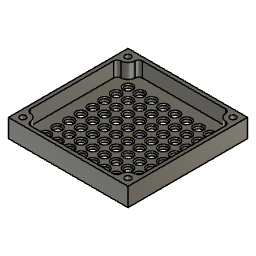
LED MATRIX GRILL (Autodesk Fusion 360 design; units mm, degrees)
Autodesk Fusion 360 part; units mm, degrees
sketch "Sketch1" plane through (0, 0, 0) normal (0, 0, 1) x (1, 0, 0)
  line L0 (32.4, 32.4) -> (-32.4, 32.4)
  line L1 (-32.4, 32.4) -> (-32.4, -32.4)
  line L2 (-32.4, -32.4) -> (32.4, -32.4)
  line L3 (32.4, -32.4) -> (32.4, 32.4)
  line L4 (32.4, 32.4) -> (-32.4, -32.4) construction
  line L5 (-32.4, 32.4) -> (32.4, -32.4) construction
  line L6 (28.5, -28.5) -> (-28.5, -28.5)
  line L7 (-28.5, -28.5) -> (-28.5, 28.5)
  line L8 (-28.5, 28.5) -> (28.5, 28.5)
  line L9 (28.5, 28.5) -> (28.5, -28.5)
  line L10 (28.5, -28.5) -> (-28.5, 28.5) construction
  circle A0 centre (28.5, 28.5) radius 1.6
  circle A1 centre (-28.5, 28.5) radius 1.6
  circle A2 centre (-28.5, -28.5) radius 1.6
  circle A3 centre (28.5, -28.5) radius 1.6
  line L11 (25.6, 25.6) -> (-25.6, 25.6)
  line L12 (-25.6, 25.6) -> (-25.6, -25.6)
  line L13 (-25.6, -25.6) -> (25.6, -25.6)
  line L14 (25.6, -25.6) -> (25.6, 25.6)
  line L15 (25.6, 25.6) -> (-25.6, -25.6) construction
  line L16 (-25.6, 25.6) -> (25.6, -25.6) construction
  line L17 (22.2, 22.2) -> (-22.2, -22.2) construction
  line L18 (-22.2, 22.2) -> (22.2, -22.2) construction
  line L19 (15.9, 15.9) -> (-15.9, -15.9) construction
  line L20 (-15.9, 15.9) -> (15.9, -15.9) construction
  line L21 (22.3, 22.3) -> (-22.3, 22.3)
  line L22 (-22.3, 22.3) -> (-22.3, -22.3)
  line L23 (-22.3, -22.3) -> (22.3, -22.3)
  line L24 (22.3, -22.3) -> (22.3, 22.3)
  line L25 (22.3, 22.3) -> (-22.3, -22.3) construction
  line L26 (-22.3, 22.3) -> (22.3, -22.3) construction
  line L27 (-22.3, 22.3) -> (-15.9286, 22.3)
  line L28 (-15.9286, 22.3) -> (-15.9286, -22.3)
  line L29 (-15.9286, -22.3) -> (-22.3, -22.3)
  line L30 (-22.3, -22.3) -> (-22.3, 22.3)
  line L31 (-15.9286, 22.3) -> (-9.5571, 22.3)
  line L32 (-9.5571, 22.3) -> (-9.5571, -22.3)
  line L33 (-9.5571, -22.3) -> (-15.9286, -22.3)
  line L34 (-15.9286, -22.3) -> (-15.9286, 22.3)
  line L35 (-9.5571, 22.3) -> (-3.1857, 22.3)
  line L36 (-3.1857, 22.3) -> (-3.1857, -22.3)
  line L37 (-3.1857, -22.3) -> (-9.5571, -22.3)
  line L38 (-9.5571, -22.3) -> (-9.5571, 22.3)
  line L39 (-3.1857, 22.3) -> (3.1857, 22.3)
  line L40 (3.1857, 22.3) -> (3.1857, -22.3)
  line L41 (3.1857, -22.3) -> (-3.1857, -22.3)
  line L42 (-3.1857, -22.3) -> (-3.1857, 22.3)
  line L43 (3.1857, 22.3) -> (9.5571, 22.3)
  line L44 (9.5571, 22.3) -> (9.5571, -22.3)
  line L45 (9.5571, -22.3) -> (3.1857, -22.3)
  line L46 (3.1857, -22.3) -> (3.1857, 22.3)
  line L47 (9.5571, 22.3) -> (15.9286, 22.3)
  line L48 (15.9286, 22.3) -> (15.9286, -22.3)
  line L49 (15.9286, -22.3) -> (9.5571, -22.3)
  line L50 (9.5571, -22.3) -> (9.5571, 22.3)
  line L51 (22.3, 22.3) -> (-22.3, 22.3)
  line L52 (-22.3, 22.3) -> (-22.3, 15.9286)
  line L53 (-22.3, 15.9286) -> (22.3, 15.9286)
  line L54 (22.3, 15.9286) -> (22.3, 22.3)
  line L55 (-22.3, 15.9286) -> (22.3, 15.9286)
  line L56 (22.3, 15.9286) -> (22.3, 9.5571)
  line L57 (22.3, 9.5571) -> (-22.3, 9.5571)
  line L58 (-22.3, 9.5571) -> (-22.3, 15.9286)
  line L59 (-22.3, 9.5571) -> (22.3, 9.5571)
  line L60 (22.3, 9.5571) -> (22.3, 3.1857)
  line L61 (22.3, 3.1857) -> (-22.3, 3.1857)
  line L62 (-22.3, 3.1857) -> (-22.3, 9.5571)
  line L63 (-22.3, 3.1857) -> (22.3, 3.1857)
  line L64 (22.3, 3.1857) -> (22.3, -3.1857)
  line L65 (22.3, -3.1857) -> (-22.3, -3.1857)
  line L66 (-22.3, -3.1857) -> (-22.3, 3.1857)
  line L67 (-22.3, -3.1857) -> (22.3, -3.1857)
  line L68 (22.3, -3.1857) -> (22.3, -9.5571)
  line L69 (22.3, -9.5571) -> (-22.3, -9.5571)
  line L70 (-22.3, -9.5571) -> (-22.3, -3.1857)
  line L71 (-22.3, -9.5571) -> (22.3, -9.5571)
  line L72 (22.3, -9.5571) -> (22.3, -15.9286)
  line L73 (22.3, -15.9286) -> (-22.3, -15.9286)
  line L74 (-22.3, -15.9286) -> (-22.3, -9.5571)
  circle A4 centre (-22.2, 22.2) radius 2
  circle A5 centre (-15.9286, 22.3) radius 2
  circle A6 centre (-9.5571, 22.3) radius 2
  circle A7 centre (-3.1857, 22.3) radius 2
  circle A8 centre (3.1857, 22.3) radius 2
  circle A9 centre (9.5571, 22.3) radius 2
  circle A10 centre (15.9286, 22.3) radius 2
  circle A11 centre (22.2, 22.2) radius 2
  circle A12 centre (-22.3, 15.9286) radius 2
  circle A13 centre (-15.9286, 15.9286) radius 2
  circle A14 centre (-9.5571, 15.9286) radius 2
  circle A15 centre (-3.1857, 15.9286) radius 2
  circle A16 centre (3.1857, 15.9286) radius 2
  circle A17 centre (9.5571, 15.9286) radius 2
  circle A18 centre (15.9286, 15.9286) radius 2
  circle A19 centre (22.3, 15.9286) radius 2
  circle A20 centre (22.3, 9.5571) radius 2
  circle A21 centre (15.9286, 9.5571) radius 2
  circle A22 centre (9.5571, 9.5571) radius 2
  circle A23 centre (3.1857, 9.5571) radius 2
  circle A24 centre (-3.1857, 9.5571) radius 2
  circle A25 centre (-9.5571, 9.5571) radius 2
  circle A26 centre (-15.9286, 9.5571) radius 2
  circle A27 centre (-22.3, 9.5571) radius 2
  circle A28 centre (-22.3, 3.1857) radius 2
  circle A29 centre (-15.9286, 3.1857) radius 2
  circle A30 centre (-9.5571, 3.1857) radius 2
  circle A31 centre (-3.1857, 3.1857) radius 2
  circle A32 centre (3.1857, 3.1857) radius 2
  circle A33 centre (9.5571, 3.1857) radius 2
  circle A34 centre (15.9286, 3.1857) radius 2
  circle A35 centre (22.3, 3.1857) radius 2
  circle A36 centre (22.3, -3.1857) radius 2
  circle A37 centre (15.9286, -3.1857) radius 2
  circle A38 centre (9.5571, -3.1857) radius 2
  circle A39 centre (3.1857, -3.1857) radius 2
  circle A40 centre (-3.1857, -3.1857) radius 2
  circle A41 centre (-9.5571, -3.1857) radius 2
  circle A42 centre (-15.9286, -3.1857) radius 2
  circle A43 centre (-22.3, -3.1857) radius 2
  circle A44 centre (-22.3, -9.5571) radius 2
  circle A45 centre (-15.9286, -9.5571) radius 2
  circle A46 centre (-9.5571, -9.5571) radius 2
  circle A47 centre (-3.1857, -9.5571) radius 2
  circle A48 centre (3.1857, -9.5571) radius 2
  circle A49 centre (9.5497, -9.5497) radius 2
  circle A50 centre (15.9286, -9.5571) radius 2
  circle A51 centre (22.3, -9.5571) radius 2
  circle A52 centre (-22.3, -15.9286) radius 2
  circle A53 centre (-22.3, -22.3) radius 2
  circle A54 centre (-15.9286, -22.3) radius 2
  circle A55 centre (-15.9286, -15.9286) radius 2
  circle A56 centre (-9.5571, -15.9286) radius 2
  circle A57 centre (-9.5571, -22.3) radius 2
  circle A58 centre (-3.1857, -15.9286) radius 2
  circle A59 centre (-3.1857, -22.3) radius 2
  circle A60 centre (3.1857, -15.9286) radius 2
  circle A61 centre (3.1857, -22.3) radius 2
  circle A62 centre (9.5571, -15.9286) radius 2
  circle A63 centre (9.5571, -22.3) radius 2
  circle A64 centre (15.9314, -15.9314) radius 2
  circle A65 centre (15.9286, -22.3) radius 2
  circle A66 centre (22.3, -15.9286) radius 2
  circle A67 centre (22.3, -22.3) radius 2
  dimension "d1" = 64.8
  dimension "d2" = 64.8
  dimension "d3" = 57
  dimension "d4" = 57
  dimension "d5" = 3.2
  dimension "d6" = 3.2
  dimension "d7" = 3.2
  dimension "d8" = 3.2
  dimension "d9" = 51.2
  dimension "d10" = 51.2
  dimension "d11" = 44.4
  dimension "d12" = 44.4
  dimension "d15" = 44.6
  dimension "d16" = 44.6
  dimension "d17" = 6.3714
  dimension "d18" = 44.6
  dimension "d19" = 6.3714
  dimension "d20" = 6.3714
  dimension "d21" = 6.3714
  dimension "d22" = 6.3714
  dimension "d23" = 6.3714
  dimension "d24" = 6.3714
  dimension "d25" = 6.3714
  dimension "d26" = 6.3714
  dimension "d27" = 6.3714
  dimension "d28" = 6.3714
  dimension "d29" = 6.3714
  dimension "d30" = 4
  dimension "d31" = 4
  dimension "d32" = 4
  dimension "d33" = 4
  dimension "d34" = 4
  dimension "d35" = 4
  dimension "d36" = 4
  dimension "d37" = 4
  dimension "d38" = 4
  dimension "d39" = 4
  dimension "d40" = 4
  dimension "d41" = 4
  dimension "d42" = 4
  dimension "d43" = 4
  dimension "d44" = 4
  dimension "d45" = 4
  dimension "d46" = 4
  dimension "d47" = 4
  dimension "d48" = 4
  dimension "d49" = 4
  dimension "d50" = 4
  dimension "d51" = 4
  dimension "d52" = 4
  dimension "d53" = 4
  dimension "d54" = 4
  dimension "d55" = 4
  dimension "d56" = 4
  dimension "d57" = 4
  dimension "d58" = 4
  dimension "d59" = 4
  dimension "d60" = 4
  dimension "d61" = 4
  dimension "d62" = 4
  dimension "d63" = 4
  dimension "d64" = 4
  dimension "d65" = 4
  dimension "d66" = 4
  dimension "d67" = 4
  dimension "d68" = 4
  dimension "d69" = 4
  dimension "d70" = 4
  dimension "d71" = 4
  dimension "d72" = 4
  dimension "d73" = 4
  dimension "d74" = 4
  dimension "d75" = 4
  dimension "d76" = 4
  dimension "d77" = 4
  dimension "d78" = 4
  dimension "d79" = 4
  dimension "d80" = 4
  dimension "d81" = 4
  dimension "d82" = 4
  dimension "d83" = 4
  dimension "d84" = 4
  dimension "d85" = 4
  dimension "d86" = 4
  dimension "d87" = 4
  dimension "d88" = 4
  dimension "d89" = 4
  dimension "d90" = 4
  dimension "d91" = 4
  dimension "d92" = 4
  dimension "d93" = 4
  constraint horizontal L0
  constraint perpendicular L0 L1
  constraint parallel L0 L2
  constraint parallel L1 L3
  constraint coincident L4 origin
  constraint coincident L5 origin
  constraint horizontal L6
  constraint perpendicular L6 L7
  constraint parallel L6 L8
  constraint parallel L7 L9
  constraint coincident L10 origin
  constraint coincident L8.end L9.start
  constraint coincident L7.end L8.start
  constraint coincident L6.end L7.start
  constraint coincident L6.start L9.end
  constraint horizontal L11
  constraint perpendicular L11 L12
  constraint parallel L11 L13
  constraint parallel L12 L14
  constraint coincident L15 origin
  constraint coincident L16 origin
  constraint coincident L17 origin
  constraint coincident L18 origin
  constraint coincident L19 origin
  constraint coincident L20 origin
  constraint horizontal L21
  constraint perpendicular L21 L22
  constraint parallel L21 L23
  constraint parallel L22 L24
  constraint coincident L25 origin
  constraint coincident L26 origin
  constraint horizontal L27
  constraint vertical L28
  constraint horizontal L29
  constraint vertical L30
  constraint horizontal L31
  constraint vertical L32
  constraint horizontal L33
  constraint vertical L34
  constraint horizontal L35
  constraint vertical L36
  constraint horizontal L37
  constraint vertical L38
  constraint horizontal L39
  constraint vertical L40
  constraint horizontal L41
  constraint vertical L42
  constraint horizontal L43
  constraint vertical L44
  constraint horizontal L45
  constraint vertical L46
  constraint horizontal L47
  constraint vertical L48
  constraint horizontal L49
  constraint vertical L50
  constraint horizontal L51
  constraint vertical L52
  constraint horizontal L53
  constraint vertical L54
  constraint horizontal L55
  constraint vertical L56
  constraint horizontal L57
  constraint vertical L58
  constraint horizontal L59
  constraint vertical L60
  constraint horizontal L61
  constraint vertical L62
  constraint horizontal L63
  constraint vertical L64
  constraint horizontal L65
  constraint vertical L66
  constraint horizontal L67
  constraint vertical L68
  constraint horizontal L69
  constraint vertical L70
  constraint horizontal L71
  constraint vertical L72
  constraint horizontal L73
  constraint vertical L74
  constraint coincident L18.start A4.centre
  constraint coincident L27.end L28.start
  constraint coincident L31.end L32.start
  constraint coincident L35.end L36.start
  constraint coincident L39.end L40.start
  constraint coincident L43.end L44.start
  constraint coincident L47.end L48.start
  constraint coincident L17.start A11.centre
  constraint coincident L52.end L53.start
  constraint coincident L28 A13.centre
  constraint coincident L26 A13.centre
  constraint coincident L55 A14.centre
  constraint coincident L32 A14.centre
  constraint coincident L55 A15.centre
  constraint coincident L42 A15.centre
  constraint coincident L40 A16.centre
  constraint coincident L53 A16.centre
  constraint coincident L53 A17.centre
  constraint coincident L50 A17.centre
  constraint coincident L48 A18.centre
  constraint coincident L53 A18.centre
  constraint coincident L53.end L54.start
  constraint coincident L56.end L57.start
  constraint coincident L48 A21.centre
  constraint coincident L57 A21.centre
  constraint coincident L50 A22.centre
  constraint coincident L57 A22.centre
  constraint coincident L46 A23.centre
  constraint coincident L57 A23.centre
  constraint coincident L42 A24.centre
  constraint coincident L59 A24.centre
  constraint coincident L38 A25.centre
  constraint coincident L16 A25.centre
  constraint coincident L57 A26.centre
  constraint coincident L28 A26.centre
  constraint coincident L57.end L58.start
  constraint coincident L61.end L62.start
  constraint coincident L34 A29.centre
  constraint coincident L61 A29.centre
  constraint coincident L32 A30.centre
  constraint coincident L63 A30.centre
  constraint coincident L61 A31.centre
  constraint coincident L42 A31.centre
  constraint coincident L17 A32.centre
  constraint coincident L46 A32.centre
  constraint coincident L61 A33.centre
  constraint coincident L44 A33.centre
  constraint coincident L61 A34.centre
  constraint coincident L48 A34.centre
  constraint coincident L60.end L61.start
  constraint coincident L64.end L65.start
  constraint coincident L48 A37.centre
  constraint coincident L67 A37.centre
  constraint coincident L50 A38.centre
  constraint coincident L65 A38.centre
  constraint coincident L67 A39.centre
  constraint coincident L16 A39.centre
  constraint coincident L65 A40.centre
  constraint coincident L42 A40.centre
  constraint coincident L32 A41.centre
  constraint coincident L65 A41.centre
  constraint coincident L34 A42.centre
  constraint coincident L65 A42.centre
  constraint coincident L65.end L66.start
  constraint coincident L69.end L70.start
  constraint coincident L28 A45.centre
  constraint coincident L71 A45.centre
  constraint coincident L71 A46.centre
  constraint coincident L38 A46.centre
  constraint coincident L42 A47.centre
  constraint coincident L71 A47.centre
  constraint coincident L46 A48.centre
  constraint coincident L71 A48.centre
  constraint coincident L16 A49.centre
  constraint coincident L71 A50.centre
  constraint coincident L48 A50.centre
  constraint coincident L68.end L69.start
  constraint coincident L73.end L74.start
  constraint coincident L22.end L23.start
  constraint coincident L28.end L29.start
  constraint coincident L28 A55.centre
  constraint coincident L73 A55.centre
  constraint coincident L38 A56.centre
  constraint coincident L73 A56.centre
  constraint coincident L32.end L33.start
  constraint coincident L42 A58.centre
  constraint coincident L73 A58.centre
  constraint coincident L36.end L37.start
  constraint coincident L46 A60.centre
  constraint coincident L73 A60.centre
  constraint coincident L40.end L41.start
  constraint coincident L44 A62.centre
  constraint coincident L73 A62.centre
  constraint coincident L44.end L45.start
  constraint coincident L18 A64.centre
  constraint coincident L48.end L49.start
  constraint coincident L72.end L73.start
  constraint coincident L23.end L24.start
  measures "d1" distance of L1.end L2.end
  measures "d2" distance of L0.end L1.end
  measures "d3" distance of L7.end L8.end
  measures "d4" distance of L6.end L7.end
  measures "d5" diameter of A0
  measures "d6" diameter of A1
  measures "d7" diameter of A2
  measures "d8" diameter of A3
  measures "d9" distance of L12.end L13.end
  measures "d10" distance of L11.end L12.end
  measures "d11" distance of L17.end L18.end
  measures "d12" distance of L18.start L17.end
  measures "d15" distance of L22.end L23.end
  measures "d16" distance of L21.end L22.end
  measures "d17" distance of L21.end L27.end
  measures "d18" distance of L21.end L22.end
  measures "d19" distance of L27.end L31.end
  measures "d20" distance of L31.end L35.end
  measures "d21" distance of L35.end L39.end
  measures "d22" distance of L39.end L43.end
  measures "d23" distance of L43.end L47.end
  measures "d24" distance of L21.start L53.end
  measures "d25" distance of L52.end L57.end
  measures "d26" distance of L57.end L61.end
  measures "d27" distance of L61.end L65.end
  measures "d28" distance of L65.end L69.end
  measures "d29" distance of L69.end L73.end
  measures "d30" diameter of A4
  measures "d31" diameter of A5
  measures "d32" diameter of A6
  measures "d33" diameter of A7
  measures "d34" diameter of A8
  measures "d35" diameter of A9
  measures "d36" diameter of A10
  measures "d37" diameter of A11
  measures "d38" diameter of A12
  measures "d39" diameter of A13
  measures "d40" diameter of A14
  measures "d41" diameter of A15
  measures "d42" diameter of A16
  measures "d43" diameter of A17
  measures "d44" diameter of A18
  measures "d45" diameter of A19
  measures "d46" diameter of A20
  measures "d47" diameter of A21
  measures "d48" diameter of A22
  measures "d49" diameter of A23
  measures "d50" diameter of A24
  measures "d51" diameter of A25
  measures "d52" diameter of A26
  measures "d53" diameter of A27
  measures "d54" diameter of A28
  measures "d55" diameter of A29
  measures "d56" diameter of A30
  measures "d57" diameter of A31
  measures "d58" diameter of A32
  measures "d59" diameter of A33
  measures "d60" diameter of A34
  measures "d61" diameter of A35
  measures "d62" diameter of A36
  measures "d63" diameter of A37
  measures "d64" diameter of A38
  measures "d65" diameter of A39
  measures "d66" diameter of A40
  measures "d67" diameter of A41
  measures "d68" diameter of A42
  measures "d69" diameter of A43
  measures "d70" diameter of A44
  measures "d71" diameter of A45
  measures "d72" diameter of A46
  measures "d73" diameter of A47
  measures "d74" diameter of A48
  measures "d75" diameter of A49
  measures "d76" diameter of A50
  measures "d77" diameter of A51
  measures "d78" diameter of A52
  measures "d79" diameter of A53
  measures "d80" diameter of A54
  measures "d81" diameter of A55
  measures "d82" diameter of A56
  measures "d83" diameter of A57
  measures "d84" diameter of A58
  measures "d85" diameter of A59
  measures "d86" diameter of A60
  measures "d87" diameter of A61
  measures "d88" diameter of A62
  measures "d89" diameter of A63
  measures "d90" diameter of A64
  measures "d91" diameter of A65
  measures "d92" diameter of A66
  measures "d93" diameter of A67
extrude "Extrude1" add sketch "Sketch1" along normal blind 2 contours L0 L1 L2 L3 | L6 L7 L8 L9 A0 A1 A2 A3 | L11 L12 L13 L14 | L21 L24 L48 L51 L53 L54 L55 A10 A11 A18 A19 | L21 L44 L47 L48 L50 L51 L53 L55 A9 A10 A17 A18 | L21 L40 L43 L44 L46 L50 L51 L53 L55 A8 A9 A16 A17 | L24 L48 L53 L55 L56 L57 L59 A18 A19 A20 A21 | L44 L48 L50 L53 L55 L57 L59 A17 A18 A21 A22 | L21 L36 L39 L40 L42 L46 L51 L53 L55 A7 A8 A15 A16 | L40 L44 L46 L50 L53 L55 L57 L59 A16 A17 A22 A23 | L24 L48 L57 L59 L60 L61 L63 A20 A21 A34 A35 | L44 L48 L50 L57 L59 L61 L63 A21 A22 A33 A34 | L21 L32 L35 L36 L38 L42 L51 L53 L55 A6 A7 A14 A15 | L36 L40 L42 L46 L53 L55 L57 L59 A15 A16 A23 A24 | L40 L44 L46 L50 L57 L59 L61 L63 A22 A23 A32 A33 | L21 L28 L31 L32 L34 L38 L51 L53 L55 A5 A6 A13 A14 | L32 L36 L38 L42 L53 L55 L57 L59 A14 A15 A24 A25 | L36 L40 L42 L46 L57 L59 L61 L63 A23 A24 A31 A32 | L24 L48 L61 L63 L64 L65 L67 A34 A35 A36 A37 | L44 L48 L50 L61 L63 L65 L67 A33 A34 A37 A38 | L40 L44 L46 L50 L61 L63 L65 L67 A32 A33 A38 A39 | L21 L22 L27 L28 L30 L34 L51 L52 L53 L55 A4 A5 A12 A13 | L28 L32 L34 L38 L53 L55 L57 L59 A13 A14 A25 A26 | L32 L36 L38 L42 L57 L59 L61 L63 A24 A25 A30 A31 | L36 L40 L42 L46 L61 L63 L65 L67 A31 A32 A39 A40 | L24 L48 L65 L67 L68 L69 L71 A36 A37 A50 A51 | L44 L48 L50 L65 L67 L69 L71 A37 A38 A49 A50 | L22 L28 L30 L34 L53 L55 L57 L58 L59 A12 A13 A26 A27 | L28 L32 L34 L38 L57 L59 L61 L63 A25 A26 A29 A30 | L32 L36 L38 L42 L61 L63 L65 L67 A30 A31 A40 A41 | L40 L44 L46 L50 L65 L67 L69 L71 A38 A39 A48 A49 | L36 L40 L42 L46 L65 L67 L69 L71 A39 A40 A47 A48 | L22 L28 L30 L34 L57 L59 L61 L62 L63 A26 A27 A28 A29 | L28 L32 L34 L38 L61 L63 L65 L67 A29 A30 A41 A42 | L24 L48 L69 L71 L72 L73 A50 A51 A64 A66 | L44 L48 L50 L69 L71 L73 A49 A50 A62 A64 | L32 L36 L38 L42 L65 L67 L69 L71 A40 A41 A46 A47 | L40 L44 L46 L50 L69 L71 L73 A48 A49 A60 A62 | L22 L28 L30 L34 L61 L63 L65 L66 L67 A28 A29 A42 A43 | L28 L32 L34 L38 L65 L67 L69 L71 A41 A42 A45 A46 | L36 L40 L42 L46 L69 L71 L73 A47 A48 A58 A60 | L23 L24 L48 L73 A64 A65 A66 A67 | L23 L44 L48 L49 L50 L73 A62 A63 A64 A65 | L32 L36 L38 L42 L69 L71 L73 A46 A47 A56 A58 | L22 L28 L30 L34 L65 L67 L69 L70 L71 A42 A43 A44 A45 | L23 L40 L44 L45 L46 L50 L73 A60 A61 A62 A63 | L28 L32 L34 L38 L69 L71 L73 A45 A46 A55 A56 | L23 L36 L40 L41 L42 L46 L73 A58 A59 A60 A61 | L22 L28 L30 L34 L69 L71 L73 L74 A44 A45 A52 A55 | L23 L32 L36 L37 L38 L42 L73 A56 A57 A58 A59 | L23 L28 L32 L33 L34 L38 L73 A54 A55 A56 A57 | L22 L23 L28 L29 L30 L34 L73 A52 A53 A54 A55
sketch "Sketch2" plane through (0, 0, 2) normal (0, 0, 1) x (-1, 0, 0)
  circle A0 centre (15.9286, 15.9286) radius 2
  circle A1 centre (15.9286, 9.5571) radius 2
  circle A2 centre (15.9286, 3.1857) radius 2
  circle A3 centre (15.9286, -9.5571) radius 2
  circle A4 centre (15.9286, -3.1857) radius 2
  circle A5 centre (9.5571, -3.1857) radius 2
  circle A6 centre (-9.5571, -3.1857) radius 2
  circle A7 centre (-9.5497, 9.5497) radius 2
  circle A8 centre (-3.1857, 9.5571) radius 2
  circle A9 centre (-3.1857, 3.1857) radius 2
  circle A10 centre (-9.5571, 3.1857) radius 2
  circle A11 centre (9.5571, 9.5571) radius 2
  circle A12 centre (9.5571, 3.1857) radius 2
  circle A13 centre (3.1857, 3.1857) radius 2
  circle A14 centre (3.1857, 9.5571) radius 2
  circle A15 centre (9.5571, 15.9286) radius 2
  circle A16 centre (3.1857, 15.9286) radius 2
  circle A17 centre (-3.1857, 15.9286) radius 2
  circle A18 centre (-9.5571, 15.9286) radius 2
  circle A19 centre (-15.9314, 15.9314) radius 2
  circle A20 centre (-15.9286, 9.5571) radius 2
  circle A21 centre (-15.9286, 3.1857) radius 2
  circle A22 centre (-15.9286, -3.1857) radius 2
  circle A23 centre (-15.9286, -9.5571) radius 2
  circle A24 centre (-15.9286, -15.9286) radius 2
  circle A25 centre (-9.5571, -9.5571) radius 2
  circle A26 centre (3.1857, -3.1857) radius 2
  circle A27 centre (-3.1857, -3.1857) radius 2
  circle A28 centre (9.5571, -9.5571) radius 2
  circle A29 centre (15.9286, -15.9286) radius 2
  circle A30 centre (15.9286, -22.3) radius 2
  circle A31 centre (22.2, -22.2) radius 2
  circle A32 centre (22.3, -15.9286) radius 2
  circle A33 centre (22.3, -9.5571) radius 2
  circle A34 centre (22.3, -3.1857) radius 2
  circle A35 centre (22.3, 3.1857) radius 2
  circle A36 centre (22.3, 9.5571) radius 2
  circle A37 centre (-3.1857, -15.9286) radius 2
  circle A38 centre (9.5571, -15.9286) radius 2
  circle A39 centre (28.5, -28.5) radius 1.6
  circle A40 centre (3.1857, -22.3) radius 2
  circle A41 centre (9.5571, -22.3) radius 2
  circle A42 centre (3.1857, -15.9286) radius 2
  circle A43 centre (3.1857, -9.5571) radius 2
  circle A44 centre (-3.1857, -9.5571) radius 2
  circle A45 centre (-3.1857, -22.3) radius 2
  circle A46 centre (22.3, 22.3) radius 2
  circle A47 centre (22.3, 15.9286) radius 2
  circle A48 centre (-9.5571, -15.9286) radius 2
  circle A49 centre (-15.9286, 22.3) radius 2
  circle A50 centre (-22.3, 9.5571) radius 2
  circle A51 centre (-22.2, -22.2) radius 2
  circle A52 centre (-22.3, 22.3) radius 2
  circle A53 centre (-22.3, 15.9286) radius 2
  circle A54 centre (3.1857, 22.3) radius 2
  circle A55 centre (15.9286, 22.3) radius 2
  circle A56 centre (-3.1857, 22.3) radius 2
  circle A57 centre (-15.9286, -22.3) radius 2
  circle A58 centre (-22.3, 3.1857) radius 2
  circle A59 centre (-22.3, -15.9286) radius 2
  circle A60 centre (-22.3, -3.1857) radius 2
  circle A61 centre (-9.5571, -22.3) radius 2
  circle A62 centre (-22.3, -9.5571) radius 2
  circle A63 centre (-9.5571, 22.3) radius 2
  circle A64 centre (9.5571, 22.3) radius 2
  circle A65 centre (28.5, 28.5) radius 1.6
  circle A66 centre (-28.5, 28.5) radius 1.6
  circle A67 centre (-28.5, -28.5) radius 1.6
  line L0 (-32.4, 32.4) -> (-32.4, -32.4)
  line L1 (-32.4, -32.4) -> (32.4, -32.4)
  line L2 (32.4, -32.4) -> (32.4, 32.4)
  line L3 (32.4, 32.4) -> (-32.4, 32.4)
  line L4 (32.4, -32.4) -> (-32.4, -32.4)
  line L5 (-32.4, -32.4) -> (-32.4, 32.4)
  line L6 (-32.4, 32.4) -> (32.4, 32.4)
  line L7 (32.4, 32.4) -> (32.4, -32.4)
  circle A68 centre (28.5, -28.5) radius 1.6
  circle A69 centre (-28.5, -28.5) radius 1.6
  circle A70 centre (28.5, 28.5) radius 1.6
  circle A71 centre (-28.5, 28.5) radius 1.6
  line L8 (30.4, -30.4) -> (-30.4, -30.4)
  line L9 (-30.4, -30.4) -> (-30.4, 30.4)
  line L10 (-30.4, 30.4) -> (30.4, 30.4)
  line L11 (30.4, 30.4) -> (30.4, -30.4)
  line L12 (30.4, -30.4) -> (-30.4, 30.4) construction
  line L13 (-30.4, -30.4) -> (30.4, 30.4) construction
  circle A72 centre (28.5, -28.5) radius 3.9
  circle A73 centre (-28.5, -28.5) radius 3.9
  circle A74 centre (28.5, 28.5) radius 3.9
  circle A75 centre (-28.5, 28.5) radius 3.9
  dimension "d96" = 3.2
  dimension "d97" = 3.2
  dimension "d98" = 3.2
  dimension "d99" = 3.2
  dimension "d100" = 60.8
  dimension "d101" = 60.8
  constraint horizontal L4
  constraint vertical L5
  constraint horizontal L6
  constraint vertical L7
  constraint coincident L0.start L3.end
  constraint coincident L1.end L2.start
  constraint concentric A39 A68
  constraint concentric A67 A69
  constraint concentric A65 A70
  constraint concentric A66 A71
  constraint horizontal L8
  constraint perpendicular L8 L9
  constraint parallel L8 L10
  constraint parallel L9 L11
  constraint coincident L12 origin
  constraint coincident L13 origin
  constraint concentric A68 A72
  constraint tangent L1 A72
  constraint concentric A69 A73
  constraint tangent L1 A73
  constraint concentric A70 A74
  constraint tangent L3 A74
  constraint concentric A66 A75
  constraint tangent L3 A75
  measures "d96" diameter of A68
  measures "d97" diameter of A69
  measures "d98" diameter of A70
  measures "d99" diameter of A71
  measures "d100" distance of L9.end L10.end
  measures "d101" distance of L8.end L9.end
extrude "Extrude2" add sketch "Sketch2" along normal blind 8 contours L0 L3 L5 L6 A75 | L0 L5 L9 A73 A75 | L9 L10 A75 | L3 L6 L10 A74 A75 | L0 L1 L4 L5 A73 | L8 L9 A73 | L9 L10 A75 | L2 L3 L6 L7 A74 | L10 L11 A74 | L8 L9 A73 | L1 L4 L8 A72 A73 | L2 L7 L11 A72 A74 | L10 L11 A74 | L1 L2 L4 L7 A72 | L8 L11 A72 | L8 L11 A72
fillet "Fillet1" radius 2 8 edges at (30.4, 25.0941, 6) (25.0941, 30.4, 6) (-25.0941, 30.4, 6) (-30.4, 25.0941, 6) (-30.4, -25.0941, 6) (-25.0941, -30.4, 6) (25.0941, -30.4, 6) (30.4, -25.0941, 6)
chamfer "Chamfer1" distance 0.6 angle 45 16 edges at (20.4353, -21.5768, 2) (14.0639, -21.5768, 2) (7.6925, -21.5768, 2) (1.3211, -21.5768, 2) (-5.0504, -21.5768, 2) (-11.4218, -21.5768, 2) (-17.7932, -21.5768, 2) (-24.1647, -21.5768, 2) (-24.1647, -15.2053, 2) (-17.7932, -15.2053, 2) (-11.4218, -15.2053, 2) (-5.0504, -15.2053, 2) (1.3211, -15.2053, 2) (7.6925, -15.2053, 2) (14.0667, -15.2081, 2) (20.4353, -15.2053, 2)
chamfer "Chamfer2" distance 0.6 angle 45 16 edges at (20.4353, -8.8339, 2) (14.0639, -8.8339, 2) (7.685, -8.8265, 2) (1.3211, -8.8339, 2) (-5.0504, -8.8339, 2) (-11.4218, -8.8339, 2) (-17.7932, -8.8339, 2) (-24.1647, -8.8339, 2) (-24.1647, -2.4625, 2) (-17.7932, -2.4625, 2) (-11.4218, -2.4625, 2) (-5.0504, -2.4625, 2) (1.3211, -2.4625, 2) (7.6925, -2.4625, 2) (14.0639, -2.4625, 2) (20.4353, -2.4625, 2)
chamfer "Chamfer3" distance 0.6 angle 45 32 edges at (20.4353, 3.9089, 2) (20.4353, 10.2804, 2) (20.4353, 16.6518, 2) (20.3353, 22.9232, 2) (14.0639, 23.0232, 2) (14.0639, 16.6518, 2) (14.0639, 10.2804, 2) (14.0639, 3.9089, 2) (7.6925, 3.9089, 2) (7.6925, 10.2804, 2) (7.6925, 16.6518, 2) (7.6925, 23.0232, 2) (1.3211, 23.0232, 2) (1.3211, 16.6518, 2) (1.3211, 10.2804, 2) (1.3211, 3.9089, 2) (-5.0504, 3.9089, 2) (-5.0504, 10.2804, 2) (-5.0504, 16.6518, 2) (-5.0504, 23.0232, 2) (-11.4218, 23.0232, 2) (-11.4218, 16.6518, 2) (-11.4218, 10.2804, 2) (-11.4218, 3.9089, 2) (-17.7932, 3.9089, 2) (-17.7932, 10.2804, 2) (-17.7932, 16.6518, 2) (-17.7932, 23.0232, 2) (-24.0647, 22.9232, 2) (-24.1647, 16.6518, 2) (-24.1647, 10.2804, 2) (-24.1647, 3.9089, 2)
